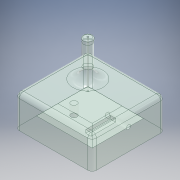
# Autodesk Inventor part: DAQcapsule
Saved by Autodesk Inventor 2018 (Build 220112000, 112)
## iProperties
Created: 2020-03-04
Part Number: DAQcapsule
Material: Generic
Document SubType Name: Modeling
Designer: Ivan
Density: 1 g/cm^3
Appearance: Default
Author: Ivan
Autodesk Inventor part; units mm, degrees
ref_plane "YZ Plane" through (0, 0, 0) normal (1, 0, 0) x (0, 1, 0)
ref_plane "XZ Plane" through (0, 0, 0) normal (0, 1, 0) x (-1, 0, 0)
ref_plane "XY Plane" through (0, 0, 0) normal (0, 0, 1) x (1, 0, 0)
sketch "Sketch1" plane through (0, 0, 0) normal (0, 0, 1) x (1, 0, 0)
  line L0 (0, 0) -> (36, 0)
  line L1 (36, 0) -> (36, 34)
  line L2 (36, 34) -> (0, 34)
  line L3 (0, 34) -> (0, 0)
  dimension "d0" = 36
  dimension "d1" = 34
  constraints: 8 end point, 2 parallel, 1 horizontal, 1 perpendicular
  measures "d0" distance of L2.end L1.end
  measures "d1" distance of L1.end L0.end
extrude "Extrusion1" add sketch "Sketch1" along normal blind 5
sketch "Sketch2" plane through (0, 0, 5) normal (0, 0, 1) x (1, 0, 0)
  circle A0 centre (13.5, 14) radius 1.4
  line L0 (0, 0) -> (36, 0) projected
  line L1 (0, 34) -> (0, 0) projected
  dimension "d6" = 2.8
  dimension "d7" = 14
  dimension "d8" = 13.5
  constraints: 1 centre point
  measures "d6" diameter of A0
  measures "d7" distance from line of L0 A0.centre
  measures "d8" distance from line of L1 A0.centre
extrude "Extrusion2" add sketch "Sketch2" along normal blind 5
sketch "Sketch3" plane through (0, 0, 5) normal (0, 0, 1) x (1, 0, 0)
  line L0 (22, 11) -> (24.5, 11)
  line L1 (24.5, 11) -> (24.5, 22.5)
  line L2 (24.5, 22.5) -> (22, 22.5)
  line L3 (22, 22.5) -> (22, 11)
  line L4 (0, 0) -> (36, 0) projected
  line L5 (0, 34) -> (0, 0) projected
  dimension "d9" = 2.5
  dimension "d10" = 11.5
  dimension "d11" = 11
  dimension "d12" = 22
  constraints: 8 end point, 2 parallel, 1 horizontal, 1 perpendicular
  measures "d9" distance of L2.end L1.end
  measures "d10" distance of L1.end L0.end
  measures "d11" distance between parallel lines of L4 L0
  measures "d12" distance between parallel lines of L5 L3
extrude "Extrusion3" cut sketch "Sketch3" against normal blind 1.5
sketch "Sketch4" plane through (0, 0, 5) normal (0, 0, 1) x (1, 0, 0)
  line L0 (0, 34) -> (36, 34)
  line L1 (36, 34) -> (36, 29)
  line L2 (36, 29) -> (0, 29)
  line L3 (0, 29) -> (0, 34)
  line L4 (36, 0) -> (36, 34) construction
  line L5 (36, 29) -> (31, 29)
  line L6 (31, 29) -> (31, 0)
  line L7 (31, 0) -> (36, 0)
  line L8 (36, 0) -> (36, 29)
  line L9 (0, 0) -> (36, 0) projected
  line L10 (31, 0) -> (0, 0)
  line L11 (0, 0) -> (0, 5)
  line L12 (0, 5) -> (31, 5)
  line L13 (31, 5) -> (31, 0)
  line L14 (0, 34) -> (0, 0) projected
  line L15 (0, 5) -> (5, 5)
  line L16 (5, 5) -> (5, 29)
  line L17 (5, 29) -> (0, 29)
  line L18 (0, 29) -> (0, 5)
  dimension "d16" = 5
  dimension "d17" = 5
  dimension "d18" = 5
  dimension "d19" = 5
  constraints: 32 end point, 8 parallel, 4 collinear, 4 horizontal, 4 perpendicular
  measures "d16" distance of L0.end L1.end
  measures "d17" distance between parallel lines of L4 L6
  measures "d18" distance between parallel lines of L12 L9
  measures "d19" distance between parallel lines of L16 L18
extrude "Extrusion4" add sketch "Sketch4" along normal blind 5 contours L0 L1 L2 L3 | L2 L16 L12 L14 | L8 L7 L6 L2 | L12 L6 L9 L11
sketch "Sketch5" plane through (0, 0, 10) normal (0, 0, 1) x (1, 0, 0)
  line L0 (0, 34) -> (36, 34)
  line L1 (36, 34) -> (36, 0)
  line L2 (36, 0) -> (0, 0)
  line L3 (0, 0) -> (0, 34)
  line L4 (36, 34) -> (0, 34) projected
  line L5 (36, 0) -> (36, 34) projected
  line L6 (0, 0) -> (36, 0) projected
  line L7 (0, 34) -> (0, 0) projected
  constraints: 8 end point, 4 collinear, 2 parallel, 1 horizontal, 1 perpendicular
extrude "Extrusion5" add sketch "Sketch5" along normal blind 5
chamfer "Chamfer1" distance 5 angle 45 4 edges at (31, 17, 10) (5, 17, 10) (18, 5, 10) (18, 29, 10)
sketch "Sketch9" plane through (36, 0, 0) normal (1, 0, 0) x (0, 0, -1)
  circle A0 centre (-10, 17) radius 1
  line L0 (-15, 0) -> (-15, 34) projected
  line L1 (-10, 10) -> (-10, 24) projected
  point P0 (0, 0)
  point P1 (-15, 17)
  point P2 (-10, 17)
  dimension "d36" = 2
  constraints: 2 midpoint, 1 centre point, 1 coincident, 1 horizontal alignment
  measures "d36" diameter of A0
extrude "Extrusion9" cut sketch "Sketch9" against normal blind 10
fillet "Fillet1" radius 2 8 edges at (36, 0, 7.5) (0, 0, 7.5) (36, 17, 15) (36, 34, 7.5) (0, 34, 7.5) (18, 34, 15) (0, 17, 15) (18, 0, 15)
sketch "Sketch10" plane through (0, 0, 15) normal (0, 0, 1) x (1, 0, 0)
  circle A0 centre (12, 22) radius 2
  line L0 (26, 24) -> (10, 24) construction
  line L1 (10, 24) -> (10, 10) construction
  point P0 (0, 0)
  dimension "d40" = 4
  constraints: 2 tangent, 1 centre point
  measures "d40" diameter of A0
extrude "Extrusion10" add sketch "Sketch10" along normal blind 15
sketch "Sketch11" plane through (0, 0, 15) normal (0, 0, 1) x (1, 0, 0)
  circle A0 centre (12, 22) radius 2 construction
  circle A1 centre (12, 22) radius 0.375
  point P0 (0, 0)
  dimension "d43" = 0.75
  constraints: 1 centre point, 1 coincident
  measures "d43" diameter of A1
extrude "Extrusion12" cut sketch "Sketch11" against normal blind 5
fillet "Fillet2" radius 5 1 edges at (10, 22, 15)
ref_plane "Work Plane1" through (12, 22, 32) normal (0, 0, 1) x (1, 0, 0)
sketch "Sketch13" plane through (12, 22, 32) normal (0, 0, 1) x (1, 0, 0)
  circle A0 centre (0, 0) radius 2.25
  point P0 (-12, -22)
  dimension "d50" = 4.5
  constraints: 1 centre point, 1 coincident
  measures "d50" diameter of A0
loft "Loft1" add profiles "Sketch13" section 2 edges at (10, 22, 30)
extrude "Extrusion13" cut sketch "Sketch11" along normal up to surface (17 mm away)
fillet "Fillet3" radius 0.5 1 edges at (9.75, 22, 32)
equation "\"d17\" = d16"
equation "\"d18\" = d16"
equation "\"d19\" = d16"
body "Solid1"
